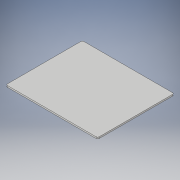
# Autodesk Inventor part: ControllerPCB
Saved by Autodesk Inventor 2018.3 (Build 223284000, 284)
## iProperties
Created: 2018-09-03
Part Number: ControllerPCB
Material: Generisch
Document SubType Name: Modeling
Designer: JochenAlt
Density: 1 g/cm^3
Appearance: Vorgabe
Author: JochenAlt
Autodesk Inventor part; units mm, degrees
ref_plane "YZ Plane" through (0, 0, 0) normal (1, 0, 0) x (0, 1, 0)
ref_plane "XZ Plane" through (0, 0, 0) normal (0, 1, 0) x (-1, 0, 0)
ref_plane "XY Plane" through (0, 0, 0) normal (0, 0, 1) x (1, 0, 0)
sketch "Skizze1" plane through (0, 0, 0) normal (0, 0, 1) x (1, 0, 0)
  line L0 (0, -70.5799) -> (0, 70.5799) construction
  line L1 (-84.5799, 0) -> (84.5799, 0) construction
  line L2 (-58, 50) -> (58, 50)
  line L3 (60, 48) -> (60, -48)
  line L4 (58, -50) -> (-58, -50)
  line L5 (-60, -48) -> (-60, 48)
  arc A0 (-60, -48) -> (-58, -50) centre (-58, -48) ccw
  arc A1 (58, -50) -> (60, -48) centre (58, -48) ccw
  arc A2 (60, 48) -> (58, 50) centre (58, 48) ccw
  arc A3 (-58, 50) -> (-60, 48) centre (-58, 48) ccw
  point P0 (0, 0)
  point P1 (-60, 50)
  point P2 (60, -50)
  point P3 (60, 50)
  point P4 (-60, -50)
  dimension "d14" = 120
  dimension "d15" = 100
  dimension "d16" = 2
  constraints: 8 end point, 8 point on circle, 8 point on line, 8 tangent, 4 centre point, 3 equal radius, 2 parallel, 1 horizontal, 1 perpendicular, 2 other
  measures "d14" distance of point (60, -50) point (-60, -50)
  measures "d15" distance of point (60, 50) point (60, -50)
  measures "d16" radius of A0
extrude "Extrusion1" add sketch "Skizze1" along normal blind 2
